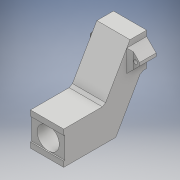
# Autodesk Inventor part: RescueKit-Pipev3
Saved by Autodesk Inventor 2018 (Build 220112000, 112)
## iProperties
Created: 2019-03-13
Part Number: RescueKit-Pipev3
Material: 一般
Document SubType Name: Modeling
Designer: shun2
Density: 1 g/cm^3
Appearance: 既定
Author: shun2
Autodesk Inventor part; units mm, degrees
ref_plane "YZ Plane" through (0, 0, 0) normal (1, 0, 0) x (0, 1, 0)
ref_plane "XZ Plane" through (0, 0, 0) normal (0, 1, 0) x (-1, 0, 0)
ref_plane "XY Plane" through (0, 0, 0) normal (0, 0, 1) x (1, 0, 0)
sketch "スケッチ1" plane through (0, 0, 0) normal (1, 0, 0) x (0, 1, 0)
  line L0 (0, -20) -> (0, 0)
  line L1 (-10, 0) -> (18.2843, 0) construction
  line L2 (-10, 0) -> (34.366, 0) construction
  line L3 (-75, -65) -> (-27.8868, -65)
  line L4 (-38.094, -35) -> (-75, -35)
  line L5 (-75, -35) -> (-75, -65)
  line L6 (0, 5) -> (-15, 5)
  line L7 (0, -25) -> (0, 5)
  line L8 (-5, -25) -> (-25, -60)
  line L9 (-15, 5) -> (-38.094, -35)
  line L10 (-15, 5) -> (31.188, 5) construction
  line L11 (-25, -60) -> (-27.8868, -65)
  line L12 (-25, -60) -> (-19.2265, -60) construction
  line L13 (-5, -25) -> (0, -25)
  dimension "d23" = 120
  constraints: 28 end point, 6 horizontal, 2 equal length, 2 parallel
  measures "d23" angle of L11 L12
extrude "押し出し1" add sketch "スケッチ1" along normal blind 20
sketch "スケッチ2" plane through (20, 0, 0) normal (1, 0, 0) x (0, 0, -1)
  line L0 (0, 0) -> (0, -10) projected
  line L1 (0, -10) -> (40, -33.094) projected
  line L2 (40, -33.094) -> (40, -75) projected
  line L3 (40, -75) -> (60, -75) projected
  line L4 (60, -75) -> (60, -28.094) projected
  line L5 (60, -28.094) -> (20, -5) projected
  line L6 (20, -5) -> (20, 0) projected
  line L7 (20, 0) -> (0, 0) projected
  line L8 (65, -75) -> (65, -27.8868) projected
  line L9 (65, -27.8868) -> (60, -25) projected
  line L10 (60, -25) -> (25, -5) projected
  line L11 (25, -5) -> (25, 0) projected
  line L12 (25, 0) -> (-5, 0) projected
  line L13 (-5, 0) -> (-5, -15) projected
  line L14 (-5, -15) -> (35, -38.094) projected
  line L15 (35, -38.094) -> (35, -75) projected
  line L16 (35, -75) -> (65, -75) projected
extrude "押し出し2" cut sketch "スケッチ2" against normal blind 20 contours L0 L1 L2 L16 L15 L14 L13 L12 | L12 L11 L10 L9 L8 L16 L4 L5 L6 keep common part
sketch "スケッチ3" plane through (20, 0, 0) normal (1, 0, 0) x (0, 0, -1)
  line L0 (60, -75) -> (60, -28.094) projected
  line L1 (60, -75) -> (65, -75) projected
  line L2 (65, -75) -> (65, -27.8868) projected
  line L3 (65, -27.8868) -> (60, -25) projected
  line L4 (60, -25) -> (25, -5) projected
  line L5 (25, -5) -> (25, 0) projected
  line L6 (25, 0) -> (20, 0) projected
  line L7 (20, -5) -> (20, 0) projected
  line L8 (60, -28.094) -> (20, -5) projected
  line L9 (40, -33.094) -> (40, -75) projected
  line L10 (0, -10) -> (40, -33.094) projected
  line L11 (0, 0) -> (0, -10) projected
  line L12 (0, 0) -> (-5, 0) projected
  line L13 (-5, 0) -> (-5, -15) projected
  line L14 (-5, -15) -> (35, -38.094) projected
  line L15 (35, -38.094) -> (35, -75) projected
  line L16 (35, -75) -> (40, -75) projected
  line L17 (65, -75) -> (35, -75)
  line L18 (25, 0) -> (-5, 0)
  constraints: 4 end point, 1 horizontal, 1 parallel
extrude "押し出し3" add sketch "スケッチ3" along normal blind 5
sketch "スケッチ4" plane through (0, 0, 0) normal (-1, 0, 0) x (0, 0, 1)
  line L0 (-40, -75) -> (-40, -33.094) projected
  line L1 (-35, -75) -> (-40, -75) projected
  line L2 (-35, -38.094) -> (-35, -75) projected
  line L3 (5, -15) -> (-35, -38.094) projected
  line L4 (5, 0) -> (5, -15) projected
  line L5 (0, 0) -> (5, 0) projected
  line L6 (0, -10) -> (0, 0) projected
  line L7 (-40, -33.094) -> (0, -10) projected
  line L8 (-60, -28.094) -> (-60, -75) projected
  line L9 (-20, -5) -> (-60, -28.094) projected
  line L10 (-20, 0) -> (-20, -5) projected
  line L11 (-25, 0) -> (-20, 0) projected
  line L12 (-25, -5) -> (-25, 0) projected
  line L13 (-60, -25) -> (-25, -5) projected
  line L14 (-65, -27.8868) -> (-60, -25) projected
  line L15 (-65, -75) -> (-65, -27.8868) projected
  line L16 (-60, -75) -> (-65, -75) projected
  line L17 (-25, -5) -> (-25, 0) projected
  line L18 (5, 0) -> (-25, 0)
  line L19 (-65, -75) -> (-65, -27.8868) projected
  line L20 (-35, -75) -> (-65, -75)
  constraints: 4 end point, 2 horizontal
extrude "押し出し4" add sketch "スケッチ4" along normal blind 5
sketch "スケッチ5" plane through (25, 0, 0) normal (1, 0, 0) x (0, 0, -1)
  line L0 (65, -75) -> (65, -27.8868) projected
  line L1 (65, -27.8868) -> (60, -25) projected
  line L2 (60, -25) -> (25, -5) projected
  line L3 (25, -5) -> (25, 0) projected
  line L4 (25, 0) -> (-5, 0) projected
  line L5 (-5, 0) -> (-5, -15) projected
  line L6 (-5, -15) -> (35, -38.094) projected
  line L7 (35, -38.094) -> (35, -75) projected
  line L8 (35, -75) -> (65, -75) projected
  point P0 (0, 0)
chamfer "面取り1" distance 2 angle 45 2 edges at (10, -38.094, -35) (10, -5, -25)
sketch "スケッチ6" plane through (25, -75, -65) normal (0, -1, 0) x (1, 0, 0)
  circle A0 centre (-15, 15) radius 10
  line L0 (0, 0) -> (-30, 0) projected
  line L1 (0, 30) -> (0, 0) projected
  line L2 (-30, 30) -> (0, 30) projected
  line L3 (-30, 0) -> (-30, 30) projected
  line L4 (-25, 5) -> (-25, 25) projected
  line L5 (-5, 25) -> (-25, 25) projected
  line L6 (-5, 25) -> (-5, 5) projected
  line L7 (-25, 5) -> (-5, 5) projected
  point P0 (-25, 65)
  dimension "d31" = 20
  constraints: 1 centre point
  measures "d31" diameter of A0
extrude "押し出し5" add sketch "スケッチ6" against normal blind 40 contours L6 L7 A0 | A0 L5 L6 | A0 L4 L5 | L7 L4 A0
sketch "スケッチ7" plane through (25, 0, 5) normal (0, 1, 0) x (1, 0, 0)
  line L0 (0, 0) -> (0, 38.2679) projected
  line L1 (0, 15) -> (10, 15) construction
  line L2 (-5, 25) -> (-25, 25) projected
  line L3 (-25, 5) -> (-5, 5) projected
  line L4 (-25, 45) -> (-25, 5) projected
  circle A0 centre (-32.1887, 15) radius 1.75
  circle A1 centre (5, 15) radius 1.75
  line L5 (0, 25) -> (10, 15)
  line L6 (0, 5) -> (10, 15)
  line L7 (-30, 38.2679) -> (-30, 0) projected
  line L8 (-30, 5) -> (-37.1887, 15)
  line L9 (-30, 25) -> (-37.1887, 15)
  dimension "d37" = 3.5
  dimension "d38" = 3.5
  constraints: 10 end point, 5 point on line, 2 centre point, 1 horizontal, 1 midpoint, 1 perpendicular
  measures "d37" diameter of A0
  measures "d38" diameter of A1
extrude "押し出し6" add sketch "スケッチ7" against normal blind 15
chamfer "面取り2" distance 2 angle 45 2 edges at (-12.1887, -7.5, -10) (35, -7.5, -10)
chamfer "面取り3" distance 3 angle 45 2 edges at (-5, -15, -10) (25, -15, -10)
sketch "スケッチ8" plane through (25, -75, -65) normal (0, -1, 0) x (1, 0, 0)
  line L0 (-30, 38.2635) -> (-30, 5) projected
  line L1 (0, 25) -> (-30, 25)
  line L2 (-30, 25) -> (-30, 5)
  line L3 (-30, 5) -> (0, 5)
  line L4 (0, 5) -> (0, 25)
  point P0 (-25, 65)
  constraints: 8 end point, 2 parallel, 1 horizontal, 1 perpendicular
extrude "押し出し7" cut sketch "スケッチ8" against normal blind 1
